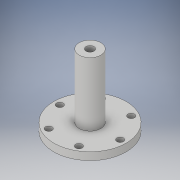
# Autodesk Inventor part: Mechanum Wheel Adapter
Saved by Autodesk Inventor 2017 (Build 210142000, 142)
## iProperties
Created: 2017-07-26
Part Number: Mechanum Wheel Adapter
Material: Generic
Document SubType Name: Modeling
Designer: User
Density: 1 g/cm^3
Appearance: Default
Author: User
Autodesk Inventor part; units mm, degrees
ref_plane "YZ Plane" through (0, 0, 0) normal (1, 0, 0) x (0, 1, 0)
ref_plane "XZ Plane" through (0, 0, 0) normal (0, 1, 0) x (-1, 0, 0)
ref_plane "XY Plane" through (0, 0, 0) normal (0, 0, 1) x (1, 0, 0)
sketch "Sketch1" plane through (0, 0, 0) normal (0, 0, 1) x (1, 0, 0)
  line L0 (0, 0) -> (0, 26.4) construction
  line L1 (3.175, 56) -> (3.175, 0)
  line L2 (28.4, 0) -> (28.4, 6)
  line L3 (3.175, 0) -> (28.4, 0)
  line L4 (8.5, 56) -> (8.5, 6)
  line L5 (8.5, 6) -> (28.4, 6)
  line L6 (8.5, 56) -> (8.5, -232.68) construction
  line L7 (8.5, 56) -> (8.5, 16.2) construction
  line L8 (8.5, 56) -> (3.175, 56)
  dimension "d0" = 26.4
  dimension "d5" = 6
  dimension "d11" = 5.325
  dimension "d32" = 3.175
  dimension "d37" = 28.4
  dimension "d38" = 50
  constraints: 18 end point, 3 vertical, 2 horizontal, 2 point on line, 1 perpendicular
  measures "d0" distance of L0.start L0.end
  measures "d5" distance of L2.start L2.end
  measures "d11" distance of L1.start L4.start
  measures "d32" distance between parallel lines of L0 L1
  measures "d37" distance between parallel lines of L0 L2
  measures "d38" distance of L4.start L4.end
revolve "Revolution1" add sketch "Sketch1" angle 360 about axis through (0, 0, 0) along (0, 1, 0)
sketch "Sketch4" plane through (0, 6, 0) normal (0, 1, 0) x (1, 0, 0)
  line L0 (0, 0) -> (-23.75, 0) construction
  circle A0 centre (-23.75, 0) radius 2.6
  circle A1 centre (-11.875, -20.5681) radius 2.6
  circle A2 centre (11.875, -20.5681) radius 2.6
  circle A3 centre (23.75, 0) radius 2.6
  circle A4 centre (11.875, 20.5681) radius 2.6
  circle A5 centre (-11.875, 20.5681) radius 2.6
  dimension "d23" = 23.75
  dimension "d24" = 5.2
  dimension "d27" = 360
  constraints: 6 centre point, 2 end point, 1 coincident, 1 horizontal, 13 other
  measures "d23" distance of L0.start L0.end
  measures "d24" diameter of A0
extrude "Extrusion1" cut sketch "Sketch4" against normal blind 6
sketch "Sketch5" plane through (0, 0, 0) normal (0, -1, 0) x (1, 0, 0)
  circle A0 centre (0, 0) radius 3.175 projected
  line L0 (0, 0) -> (6.9148, -6.9148)
  line L1 (0, 0) -> (9.779, 0) construction
  dimension "d39" = 9.779
  dimension "d40" = 45
  constraints: 4 end point, 1 coincident, 1 equal length, 1 horizontal
  measures "d39" distance of L0.start L0.end
  measures "d40" angle of L0 L1
hole "Hole2" at (6.9148, 0, -6.9148) direction (0, 1, 0) diameter 2.6416 depth 5.08 tip angle 118 thread size "6-32 UNC" class "2B" standard "ANSI Unified Screw Threads"
pattern_circular "Circular Pattern1" count 4 over 360 about axis through (0, 28, 0) along (0, -1, 0) of "Hole2"
body "Solid1"
